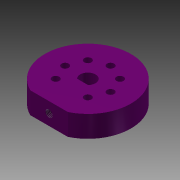
# Autodesk Inventor part: EncoderWheelInterface
Saved by Autodesk Inventor 2014 SP1 (Build 180222100, 222)
## iProperties
Created: 2015-03-21
Part Number: EncoderWheelInterface
Material: Polyethylene, High Density
Document SubType Name: Modeling
Designer: david
Density: 0.952 g/cm^3
Appearance: Smooth - Off-White
Mass: 7.79186 g
Surface Area: 37.4133 cm^2
Volume: 8.18472 cm^3
EncoderWheelInterface_Thickness: 9,000 mm
EncoderWheelInterface_Diameter: 36,000 mm
Author: david
Autodesk Inventor part; units mm, degrees
ref_plane "YZ Plane" through (0, 0, 0) normal (1, 0, 0) x (0, 1, 0)
ref_plane "XZ Plane" through (0, 0, 0) normal (0, 1, 0) x (-1, 0, 0)
ref_plane "XY Plane" through (0, 0, 0) normal (0, 0, 1) x (1, 0, 0)
sketch "BodySketch" plane through (0, 0, 0) normal (0, 1, 0) x (-1, 0, 0)
  circle A0 centre (0, 0) radius 18
  dimension "EncoderWheelInterface_Diameter" = 36
  constraints: 1 centre point, 1 coincident
  measures "EncoderWheelInterface_Diameter" diameter of A0
extrude "Body" add sketch "BodySketch" along normal blind 9
sketch "FasteningHoleSketch" plane through (0, 9, 0) normal (0, 1, 0) x (1, 0, 0)
  circle A0 centre (0, 0) radius 18 projected
  circle A1 centre (0, 9.5) radius 1.5
  line L0 (0, 0) -> (0, 20.8166) construction
  circle A2 centre (-6.7175, 6.7175) radius 1.5
  circle A3 centre (-9.5, 0) radius 1.5
  circle A4 centre (-6.7175, -6.7175) radius 1.5
  circle A5 centre (0, -9.5) radius 1.5
  circle A6 centre (6.7175, -6.7175) radius 1.5
  circle A7 centre (9.5, 0) radius 1.5
  circle A8 centre (6.7175, 6.7175) radius 1.5
  dimension "d3" = 9.5
  dimension "EncoderWheelInterface_FasteningHole_Diameter" = 3
  dimension "d7" = 360
  constraints: 8 centre point, 2 end point, 1 point on line, 1 vertical, 17 other
  measures "d3" distance of L0.start A1.centre
  measures "EncoderWheelInterface_FasteningHole_Diameter" diameter of A1
sketch "ShaftHoleSketch" plane through (0, 9, 0) normal (0, 1, 0) x (1, 0, 0)
  circle A0 centre (0, 0) radius 18 projected
  arc A1 (2.3238, -2.2) -> (-2.3238, -2.2) centre (0, 0) ccw
  line L0 (-2.3238, -2.2) -> (2.3238, -2.2)
  dimension "d11" = 6.4
  dimension "d12" = 1
  constraints: 2 end point, 2 point on circle, 1 centre point, 1 coincident, 1 horizontal
  measures "d11" diameter of A1
  measures "d12" distance edge to line of A1 L0
extrude "ShaftHole" cut sketch "ShaftHoleSketch" against normal up to next contours L0 A1
extrude "FasteningHole" cut sketch "FasteningHoleSketch" against normal up to next contours A1 | A2 | A3 | A4 | A6 | A7 | A8
sketch "MeplatSketch" plane through (0, 9, 0) normal (0, 1, 0) x (1, 0, 0)
  line L0 (2.3238, -2.2) -> (-2.3238, -2.2) projected
  circle A0 centre (0, 0) radius 18 projected
  line L1 (-7.846, -16.2) -> (7.846, -16.2)
  dimension "d19" = 14
  constraints: 2 end point, 2 point on circle, 1 parallel
  measures "d19" distance between parallel lines of L0 L1
extrude "Metplat" cut sketch "MeplatSketch" against normal up to next contours L1 A0 picked at (-1.3416, -16.6481)
sketch "MeplatHoleSketch" plane through (-7.846, 9, 16.2) normal (0, 0, 1) x (1, 0, 0)
  line L0 (0, -9) -> (15.692, 0) construction
  line L1 (0, 0) -> (15.692, -9) construction
  circle A0 centre (7.846, -4.5) radius 1.5
  point P0 (7.846, -9)
  dimension "EncoderWheelInterface_MeplatHole_Diameter" = 3
  constraints: 4 end point, 1 centre point, 1 midpoint
  measures "EncoderWheelInterface_MeplatHole_Diameter" diameter of A0
extrude "MeplatHole" cut sketch "MeplatHoleSketch" against normal up to surface (14 mm away)
thread "Thread1" size "M3x0.5" class "6H" standard "ANSI Metric M Profile" full length
equation "\"d3\" = EncoderWheel_FasteningHole_DistanceToCenter"
equation "\"d11\" = Encoder_Shaft_Diameter + EncoderWheelInterface_Margin"
equation "\"d12\" = Encoder_Shaft_Meplat_Depth"
equation "\"EncoderWheelInterface_Margin\" = 0.4"
equation "\"EncoderWheel_FasteningHole_DistanceToCenter\" = 9.5"
equation "\"Encoder_Shaft_Diameter\" = 6"
equation "\"Encoder_Shaft_Meplat_Depth\" = 1"
body "Solid1"
